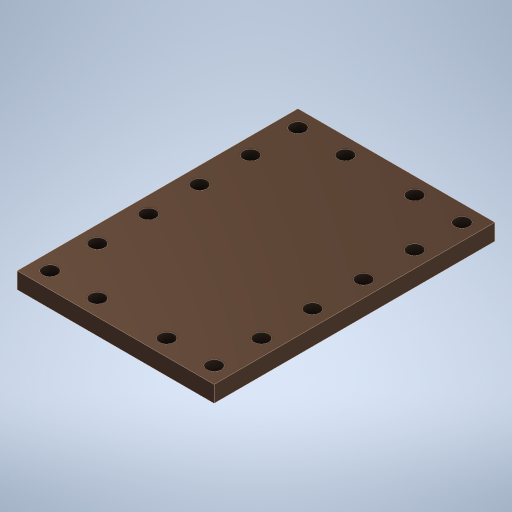
# Autodesk Inventor part: 1-35
Saved by Autodesk Inventor 2024.2 (Build 282272000, 272)
## iProperties
Created: 2024-11-02
Part Number: 1-35
Material: Bronze, Soft Tin
Document SubType Name: Modeling
Designer: Jimena Brenes
Density: 8.874 g/cm^3
Appearance: Bronze - Satin
Author: Jimena Brenes
Autodesk Inventor part; units mm, degrees
ref_plane "YZ Plane" through (0, 0, 0) normal (1, 0, 0) x (0, 1, 0)
ref_plane "XZ Plane" through (0, 0, 0) normal (0, 1, 0) x (-1, 0, 0)
ref_plane "XY Plane" through (0, 0, 0) normal (0, 0, 1) x (1, 0, 0)
sketch "Sketch1" plane through (0, 0, 0) normal (0, 1, 0) x (-1, 0, 0)
  line L0 (0, 0) -> (-54, 0)
  line L1 (-54, 0) -> (-54, -77)
  line L2 (-54, -77) -> (0, -77)
  line L3 (0, -77) -> (0, 0)
  dimension "d0" = 77
  dimension "d1" = 54
  constraints: 8 end point, 2 parallel, 1 horizontal, 1 perpendicular
  measures "d0" distance between parallel lines of L2 L0
  measures "d1" distance between parallel lines of L1 L3
extrude "Extrusion1" add sketch "Sketch1" along normal blind 4.5
sketch "Sketch2" plane through (0, 4.5, 0) normal (0, 1, 0) x (1, 0, 0)
  line L0 (4.5, 4.5) -> (49.5, 4.5) construction
  line L1 (49.5, 4.5) -> (49.5, 72.5) construction
  line L2 (49.5, 72.5) -> (4.5, 72.5) construction
  line L3 (4.5, 72.5) -> (4.5, 4.5) construction
  circle A0 centre (4.5, 4.5) radius 2
  circle A1 centre (17.5, 4.5) radius 2
  circle A2 centre (36.5, 4.5) radius 2
  circle A3 centre (49.5, 4.5) radius 2
  circle A4 centre (4.5, 17.5) radius 2
  circle A5 centre (4.5, 31.5) radius 2
  circle A6 centre (4.5, 59.5) radius 2
  circle A7 centre (4.5, 72.5) radius 2
  circle A8 centre (17.5, 72.5) radius 2
  circle A9 centre (36.5, 72.5) radius 2
  circle A10 centre (49.5, 72.5) radius 2
  circle A11 centre (49.5, 59.5) radius 2
  circle A12 centre (49.5, 45.5) radius 2
  circle A13 centre (49.5, 31.5) radius 2
  circle A14 centre (49.5, 17.5) radius 2
  line L4 (54, 0) -> (54, 77) projected
  line L5 (0, 0) -> (54, 0) projected
  line L6 (54, 77) -> (0, 77) projected
  line L7 (0, 77) -> (0, 0) projected
  circle A15 centre (4.5, 45.5) radius 2
  dimension "d4" = 4
  dimension "d5" = 4
  dimension "d6" = 4
  dimension "d7" = 4
  dimension "d8" = 4
  dimension "d9" = 4
  dimension "d11" = 4
  dimension "d12" = 4
  dimension "d13" = 4
  dimension "d14" = 4
  dimension "d15" = 4
  dimension "d16" = 4
  dimension "d17" = 4
  dimension "d18" = 4
  dimension "d19" = 4
  dimension "d20" = 4.5
  dimension "d21" = 4.5
  dimension "d22" = 4.5
  dimension "d23" = 4.5
  dimension "d24" = 13
  dimension "d25" = 14
  dimension "d26" = 13
  dimension "d27" = 4
  dimension "d28" = 14
  dimension "d29" = 13
  dimension "d30" = 19
  dimension "d31" = 13
  dimension "d32" = 14
  dimension "d33" = 14
  dimension "d34" = 14
  dimension "d35" = 13
  dimension "d36" = 19
  constraints: 16 centre point, 12 point on line, 8 end point, 4 coincident, 2 parallel, 1 horizontal, 1 perpendicular
  measures "d4" diameter of A0
  measures "d5" diameter of A1
  measures "d6" diameter of A2
  measures "d7" diameter of A3
  measures "d8" diameter of A4
  measures "d9" diameter of A5
  measures "d11" diameter of A6
  measures "d12" diameter of A7
  measures "d13" diameter of A8
  measures "d14" diameter of A9
  measures "d15" diameter of A10
  measures "d16" diameter of A11
  measures "d17" diameter of A12
  measures "d18" diameter of A13
  measures "d19" diameter of A14
  measures "d20" distance between parallel lines of L4 L1
  measures "d21" distance between parallel lines of L5 L0
  measures "d22" distance between parallel lines of L6 L2
  measures "d23" distance between parallel lines of L7 L3
  measures "d24" distance of A4.centre L0.start
  measures "d25" distance of A5.centre A4.centre
  measures "d26" distance of L2.end A6.centre
  measures "d27" diameter of A15
  measures "d28" distance of A6.centre A15.centre
  measures "d29" distance of L2.end A8.centre
  measures "d30" distance of A8.centre A9.centre
  measures "d31" distance of L1.end A11.centre
  measures "d32" distance of A12.centre A11.centre
  measures "d33" distance of A13.centre A12.centre
  measures "d34" distance of A14.centre A13.centre
  measures "d35" distance of A3.centre A2.centre
  measures "d36" distance of A1.centre A2.centre
hole "Hole1" at (4.5, 4.5, -4.5) at (17.5, 4.5, -4.5) at (4.5, 4.5, -17.5) at (36.5, 4.5, -4.5) at (4.5, 4.5, -31.5) at (49.5, 4.5, -4.5) at (49.5, 4.5, -17.5) at (4.5, 4.5, -45.5) at (4.5, 4.5, -59.5) at (4.5, 4.5, -72.5) at (17.5, 4.5, -72.5) at (36.5, 4.5, -72.5) at (49.5, 4.5, -72.5) at (49.5, 4.5, -59.5) at (49.5, 4.5, -45.5) at (49.5, 4.5, -31.5) direction (0, -1, 0) diameter 4 depth 10 tip angle 118
body "Solid1"
